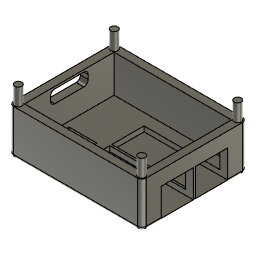
_part 2.f3cbd399-88e2-494d-b35e-1f1d8a7854d6 (Autodesk Fusion 360 design; units mm, degrees)
Autodesk Fusion 360 part; units mm, degrees
sketch "Sketch1" plane through (0, 0, 0) normal (0, 0, 1) x (1, 0, 0)
  line L0 (-15.5, 12.25) -> (15.5, 12.25)
  line L1 (15.5, 12.25) -> (15.5, -12.25)
  line L2 (15.5, -12.25) -> (-15.5, -12.25)
  line L3 (-15.5, -12.25) -> (-15.5, 12.25)
  line L4 (-15.5, 12.25) -> (15.5, -12.25) construction
  line L5 (15.5, 12.25) -> (-15.5, -12.25) construction
  dimension "d1" = 31
  dimension "d2" = 24.5
  constraint horizontal L0
  constraint perpendicular L0 L1
  constraint parallel L0 L2
  constraint parallel L1 L3
  constraint coincident L4 origin
  constraint coincident L5 origin
  measures "d1" distance of L0.start L0.end
  measures "d2" distance of L0.start L2.end
extrude "Extrude1" add sketch "Sketch1" along normal blind 10.5
shell "Shell1" thickness 1.8 removed faces 1 at (-5.1667, 4.0833, 10.5)
sketch "Sketch2" plane through (0, 0, 10.5) normal (0, 0, 1) x (-1, 0, 0)
  line L0 (13.7, 10.45) -> (13.7, -10.45)
  line L1 (13.7, -10.45) -> (-13.7, -10.45)
  line L2 (-13.7, -10.45) -> (-13.7, 10.45)
  line L3 (-13.7, 10.45) -> (13.7, 10.45)
  line L4 (15.5, 12.25) -> (-15.5, 12.25)
  line L5 (-15.5, 12.25) -> (-15.5, -12.25)
  line L6 (-15.5, -12.25) -> (15.5, -12.25)
  line L7 (15.5, -12.25) -> (15.5, 12.25)
  circle A0 centre (14.4, -11.2) radius 0.84
  line L8 (0, 0) -> (0, -2)
  line L9 (0, 0) -> (4, 0)
  circle A1 centre (-14.4, -11.2) radius 0.84
  circle A2 centre (-14.4, 11.2) radius 0.84
  circle A3 centre (14.4, 11.2) radius 0.84
  dimension "d6" = 1.68
  dimension "d7" = 11.2
  dimension "d8" = 14.4
  constraint coincident L8.start L9.start
  constraint vertical L8
  constraint perpendicular L8 L9
  constraint symmetric A0 L8 A1
  constraint symmetric A0 L9 A3
  constraint symmetric L9 A1 A2
  measures "d6" diameter of A0
  measures "d7" vertical distance of L8.start A0.centre
  measures "d8" horizontal distance of L8.start A0.centre
extrude "Extrude2" add sketch "Sketch2" along normal blind 4 contours A0 | A1 | A2 | A3
fillet "Fillet1" radius 1 1 edges at (15.5, -12.25, 5.25)
fillet "Fillet1" radius 1 1 edges at (15.5, 12.25, 5.25)
fillet "Fillet1" radius 1 1 edges at (-15.5, 12.25, 5.25)
fillet "Fillet1" radius 1 1 edges at (-15.5, -12.25, 5.25)
sketch "Sketch3" plane through (-15.5, 0, 0) normal (-1, 0, 0) x (0, -1, 0)
  line L0 (11.25, 0) -> (11.25, 10.5)
  line L1 (11.25, 10.5) -> (-11.25, 10.5)
  line L2 (-11.25, 10.5) -> (-11.25, 0)
  line L3 (-11.25, 0) -> (11.25, 0)
  line L4 (0, 0) -> (0, 7)
  line L5 (0, 7) -> (0, 8.5)
  line L6 (-3.4, 7) -> (3.4, 7)
  line L7 (4.4, 8) -> (4.4, 9)
  line L8 (3.4, 10) -> (-3.4, 10)
  line L9 (-4.4, 9) -> (-4.4, 8)
  line L10 (-4.4, 7) -> (4.4, 10) construction
  line L11 (4.4, 7) -> (-4.4, 10) construction
  arc A0 (-3.4, 10) -> (-4.4, 9) centre (-3.4, 9) ccw
  arc A1 (-4.4, 8) -> (-3.4, 7) centre (-3.4, 8) ccw
  arc A2 (3.4, 7) -> (4.4, 8) centre (3.4, 8) ccw
  arc A3 (4.4, 9) -> (3.4, 10) centre (3.4, 9) ccw
  point P0 (0, 8.5)
  dimension "d19" = 7
  dimension "d20" = 1.5
  dimension "d21" = 3
  dimension "d22" = 8.8
  dimension "d23" = 1
  constraint coincident L4.start origin
  constraint perpendicular L3 L4
  constraint parallel L4 L5
  constraint horizontal L6
  constraint perpendicular L6 L7
  constraint parallel L6 L8
  constraint parallel L7 L9
  constraint coincident L10 P0
  constraint coincident L11 P0
  constraint coincident P0 L5.end
  constraint coincident L11.end L9
  constraint coincident L11.end L8
  constraint tangent L9 A0
  constraint tangent L8 A0
  constraint coincident L10.start L9
  constraint coincident L10.start L6
  constraint tangent L9 A1
  constraint tangent L6 A1
  constraint equal A0 A1
  constraint coincident L11.start L6
  constraint coincident L11.start L7
  constraint tangent L6 A2
  constraint tangent L7 A2
  constraint equal A0 A2
  constraint coincident L10.end L7
  constraint coincident L10.end L8
  constraint tangent L7 A3
  constraint tangent L8 A3
  constraint equal A0 A3
  measures "d19" distance of L4.start L4.end
  measures "d20" distance of L4.end P0
  measures "d21" distance of L10.start L11.end
  measures "d22" distance of L10.end L11.end
  measures "d23" radius of A0
extrude "Extrude3" cut sketch "Sketch3" against normal blind 6 contours L6 L7 L8 L9 A0 A1 A2 A3
fillet "Fillet2" radius 0.75 8 edges at (-15.2071, -11.9571, 0) (-15.5, 0, 0) (-15.2071, 11.9571, 0) (0, 12.25, 0) (15.2071, 11.9571, 0) (15.5, 0, 0) (15.2071, -11.9571, 0) (0, -12.25, 0)
sketch "Sketch4" plane through (0, 0, 0) normal (0, 0, -1) x (1, 0, 0)
  arc A0 (-14.5, 11.5) -> (-14.75, 11.25) centre (-14.5, 11.25) ccw
  line L0 (-14.75, 11.25) -> (-14.75, -11.25)
  arc A1 (-14.75, -11.25) -> (-14.5, -11.5) centre (-14.5, -11.25) ccw
  line L1 (-14.5, -11.5) -> (14.5, -11.5)
  arc A2 (14.5, -11.5) -> (14.75, -11.25) centre (14.5, -11.25) ccw
  line L2 (14.75, -11.25) -> (14.75, 11.25)
  arc A3 (14.75, 11.25) -> (14.5, 11.5) centre (14.5, 11.25) ccw
  line L3 (14.5, 11.5) -> (-14.5, 11.5)
  line L4 (-14.75, 0) -> (-12.7501, 0.0149)
  line L5 (7.2499, 0.0149) -> (7.2499, 8.7649)
  line L6 (7.2499, 8.7649) -> (-12.7501, 8.7649)
  line L7 (-12.7501, 8.7649) -> (-12.7501, 0.0149)
  line L8 (7.2499, 0.0149) -> (7.2499, -8.7351)
  line L9 (7.2499, -8.7351) -> (-12.7501, -8.7351)
  line L10 (-12.7501, -8.7351) -> (-12.7501, 0.0149)
  line L11 (-12.7501, -8.7351) -> (-11.7501, -8.7351)
  line L12 (-11.7501, -8.7351) -> (-11.7501, -7.7351)
  line L13 (-11.7501, -7.7351) -> (-5.2501, -7.7351)
  line L14 (-5.2501, -7.7351) -> (-5.2501, -1.2351)
  line L15 (-5.2501, -1.2351) -> (-11.7501, -1.2351)
  line L16 (-11.7501, -1.2351) -> (-11.7501, -7.7351)
  line L17 (7.2499, 8.7649) -> (6.2499, 8.7649)
  line L18 (-5.2501, -7.7351) -> (-2.2501, -7.7351)
  line L19 (-2.2501, -7.7351) -> (12.4499, -7.7351)
  line L20 (12.4499, -7.7351) -> (12.4499, -0.7351)
  dimension "d32" = 20
  dimension "d33" = 8.75
  dimension "d34" = 1
  dimension "d35" = 1
  dimension "d38" = 6.5
  dimension "d39" = 6.5
  dimension "d42" = 1
  dimension "d54" = 3
  dimension "d55" = 14.7
  dimension "d56" = 7
  constraint midpoint L0 L4.start
  constraint vertical L5
  constraint horizontal L6
  constraint vertical L7
  constraint coincident L9 L11.end
  constraint perpendicular L10 L11
  constraint perpendicular L9 L12
  constraint horizontal L13
  constraint vertical L14
  constraint horizontal L15
  constraint vertical L16
  constraint coincident L6 L17.end
  constraint perpendicular L5 L17
  constraint perpendicular L14 L18
  constraint perpendicular L2 L19
  constraint perpendicular L19 L20
  measures "d32" distance of L5.end L6.end
  measures "d33" distance of L5.start L5.end
  measures "d34" distance of L9.end L11.end
  measures "d35" distance of L11.end L12.end
  measures "d38" distance of L12.end L13.end
  measures "d39" distance of L13.end L14.end
  measures "d42" distance of L5.end L17.end
  measures "d54" distance of L13.end L18.end
  measures "d55" distance of L18.end L19.end
  measures "d56" distance of L19.end L20.end
sketch "Sketch6" plane through (0, 0, 0) normal (0, 0, -1) x (1, 0, 0)
  arc A0 (-14.5, 11.5) -> (-14.75, 11.25) centre (-14.5, 11.25) ccw
  line L0 (-14.75, 11.25) -> (-14.75, -11.25)
  arc A1 (-14.75, -11.25) -> (-14.5, -11.5) centre (-14.5, -11.25) ccw
  line L1 (-14.5, -11.5) -> (14.5, -11.5)
  arc A2 (14.5, -11.5) -> (14.75, -11.25) centre (14.5, -11.25) ccw
  line L2 (14.75, -11.25) -> (14.75, 11.25)
  arc A3 (14.75, 11.25) -> (14.5, 11.5) centre (14.5, 11.25) ccw
  line L3 (14.5, 11.5) -> (-14.5, 11.5)
  line L4 (-15.5, 0) -> (-13.5, 0)
  line L5 (6.5, 0) -> (6.5, 8.75)
  line L6 (6.5, 8.75) -> (-13.5, 8.75)
  line L7 (-13.5, 8.75) -> (-13.5, 0)
  line L8 (-13.5, -8.75) -> (-13.5, 0)
  line L9 (6.5, -8.75) -> (-13.5, -8.75)
  line L10 (6.5, 0) -> (6.5, -8.75)
  line L11 (-13.5, 8.75) -> (-13.5, 7.75)
  line L12 (-13.5, 7.75) -> (-12.5, 7.75)
  line L13 (-12.5, 7.75) -> (-6, 7.75)
  line L14 (-6, 7.75) -> (-6, 1.25)
  line L15 (-6, 1.25) -> (-12.5, 1.25)
  line L16 (-12.5, 1.25) -> (-12.5, 7.75)
  point P0 (-13.7, 10.45)
  dimension "d57" = 2
  dimension "d58" = 10.45
  dimension "d61" = 20
  dimension "d62" = 8.75
  dimension "d63" = 1
  dimension "d64" = 1
  dimension "d65" = 6.5
  dimension "d66" = 6.5
  constraint perpendicular L0 L4
  constraint vertical L5
  constraint horizontal L6
  constraint vertical L7
  constraint symmetric L7.end L4 L8.end
  constraint symmetric L4 L5.start L10.start
  constraint symmetric L4 L5.end L9.start
  constraint symmetric L4 L6.end L8.start
  constraint coincident L7 L11.end
  constraint perpendicular L6 L11
  constraint perpendicular L7 L12
  constraint horizontal L13
  constraint vertical L14
  constraint horizontal L15
  constraint vertical L16
  measures "d57" distance of L4.start L4.end
  measures "d58" vertical distance of L4.start P0
  measures "d61" distance of L5.end L6.end
  measures "d62" distance of L5.start L5.end
  measures "d63" distance of L6.end L11.end
  measures "d64" distance of L11.end L12.end
  measures "d65" distance of L12.end L13.end
  measures "d66" distance of L12.end L15.end
extrude "Extrude5" cut sketch "Sketch6" against normal blind 9 contours L13 L14 L15 L16
sketch "Sketch7" plane through (15.5, 0, 0) normal (1, 0, 0) x (0, 1, 0)
  line L0 (-11.25, 0.75) -> (11.25, 0.75)
  line L1 (11.25, 0.75) -> (11.25, 10.5)
  line L2 (11.25, 10.5) -> (-11.25, 10.5)
  line L3 (-11.25, 10.5) -> (-11.25, 0.75)
  line L4 (0, 10.5) -> (0, 7.1)
  line L5 (-8.75, 7.1) -> (-8.75, 10.5)
  line L6 (-8.75, 7.1) -> (-7.75, 7.1)
  line L7 (-7.75, 7.1) -> (-0.25, 7.1)
  line L8 (-0.25, 7.1) -> (-0.25, 0.6)
  line L9 (-0.25, 0.6) -> (-7.75, 0.6)
  line L10 (-7.75, 0.6) -> (-7.75, 7.1)
  line L11 (0.25, 7.1) -> (0.25, 0.6)
  line L12 (0.25, 0.6) -> (7.75, 0.6)
  line L13 (7.75, 0.6) -> (7.75, 7.1)
  line L14 (7.75, 7.1) -> (0.25, 7.1)
  dimension "d69" = 3.4
  dimension "d70" = 8.75
  dimension "d73" = 1
  dimension "d74" = 7.5
  dimension "d75" = 6.5
  constraint midpoint L2 L4.start
  constraint perpendicular L2 L4
  constraint coincident L2 L5.end
  constraint perpendicular L2 L5
  constraint perpendicular L5 L6
  constraint horizontal L7
  constraint vertical L8
  constraint horizontal L9
  constraint vertical L10
  constraint symmetric L4 L6.end L13.end
  constraint symmetric L4 L7.end L11.start
  constraint symmetric L4 L8.end L11.end
  constraint symmetric L4 L9.end L12.end
  measures "d69" distance of L4.start L4.end
  measures "d70" distance of L4.end L5.start
  measures "d73" distance of L5.start L6.end
  measures "d74" distance of L8.end L9.end
  measures "d75" distance of L6.end L9.end
extrude "Extrude6" cut sketch "Sketch7" against normal blind 19.5 contours L0 L7 L8 L10 | L0 L8 L9 L10 | L0 L11 L13 L14 | L0 L11 L12 L13
